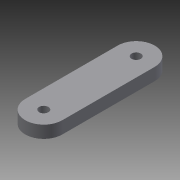
# Autodesk Inventor part: z axis arm1
Saved by Autodesk Inventor 2013 (Build 170138000, 138)
## iProperties
Created: 2017-03-09
Part Number: z axis arm1
Material: Generic
Document SubType Name: Modeling
Designer: Herman de Vries
Density: 1 g/cm^3
Author: Herman de Vries
Autodesk Inventor part; units mm, degrees
ref_plane "YZ Plane" through (0, 0, 0) normal (1, 0, 0) x (0, 1, 0)
ref_plane "XZ Plane" through (0, 0, 0) normal (0, 1, 0) x (-1, 0, 0)
ref_plane "XY Plane" through (0, 0, 0) normal (0, 0, 1) x (1, 0, 0)
sketch "Sketch1" plane through (0, 0, 0) normal (0, 0, 1) x (1, 0, 0)
  line L0 (0, 0) -> (12, 0) construction
  line L1 (12, 0) -> (12, 30)
  line L2 (12, 30) -> (0, 30) construction
  line L3 (0, 30) -> (0, 0)
  arc A0 (12, 30) -> (0, 30) centre (6, 30) ccw
  arc A1 (0, 0) -> (12, 0) centre (6, 0) ccw
  circle A2 centre (6, 30) radius 1.5
  circle A3 centre (6, 0) radius 1.5
  dimension "d0" = 12
  dimension "d1" = 30
  dimension "d2" = 3
  dimension "d3" = 3
  constraints: 8 end point, 4 centre point, 4 point on circle, 2 coincident, 2 midpoint, 2 parallel, 1 horizontal, 1 perpendicular
  measures "d0" distance of L2.end L1.end
  measures "d1" distance of L1.end L0.end
  measures "d2" diameter of A2
  measures "d3" diameter of A3
extrude "Extrusion1" add sketch "Sketch1" along normal blind 4
body "Solid1"
